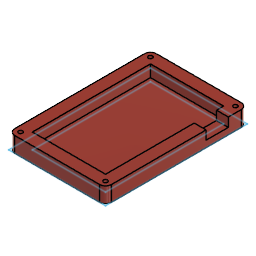
bottom_case (Autodesk Fusion 360 design; units mm, degrees)
part number: 2025-12-20-14-27-51-749
Autodesk Fusion 360 part; units mm, degrees
sketch "Schizzo1" plane through (0, 0, 0) normal (0, 0, 1) x (1, 0, 0)
  line L0 (11.1569, 43.4423) -> (72.6969, 43.4423)
  line L1 (72.6969, 43.4423) -> (72.6969, -55.9077)
  line L2 (72.6969, -55.9077) -> (11.1569, -55.9077)
  line L3 (11.1569, -55.9077) -> (11.1569, 43.4423)
  line L4 (1.157, 53.442) -> (82.697, 53.442)
  line L5 (82.697, 53.442) -> (82.697, -65.908)
  line L6 (82.697, -65.908) -> (1.157, -65.908)
  line L7 (1.157, -65.908) -> (1.157, 53.442)
  dimension "d1" = 99.35
  dimension "d2" = 61.54
  dimension "d3" = 81.54
  dimension "d4" = 119.35
  constraint horizontal L0
  constraint vertical L1
  constraint horizontal L2
  constraint vertical L3
  constraint horizontal L4
  constraint vertical L5
  constraint horizontal L6
  constraint vertical L7
  measures "d1" distance of L0.start L2.end
  measures "d2" distance of L1.end L2.end
  measures "d3" distance of L4.start L4.end
  measures "d4" distance of L4.start L6.end
sketch "Schizzo2" plane through (0, 0, 0) normal (0, 0, 1) x (1, 0, 0)
  circle A0 centre (6.1575, -60.9075) radius 1.7
  circle A1 centre (77.6967, -60.908) radius 1.7
  circle A2 centre (77.6975, 48.4425) radius 1.7
  circle A3 centre (6.1571, 48.442) radius 1.7
  circle A4 centre (6.1575, -60.9075) radius 3
  circle A5 centre (77.6967, -60.908) radius 3
  circle A6 centre (77.6975, 48.4425) radius 3
  circle A7 centre (6.1571, 48.442) radius 3
  dimension "d12" = 3.4
  dimension "d13" = 3.4
  dimension "d18" = 3.4
  dimension "d19" = 3.4
  dimension "d22" = 6
  dimension "d23" = 6
  dimension "d24" = 6
  dimension "d25" = 6
  constraint concentric A0 A4
  constraint concentric A1 A5
  constraint concentric A2 A6
  constraint concentric A3 A7
  measures "d12" diameter of A0
  measures "d13" diameter of A1
  measures "d18" diameter of A2
  measures "d19" diameter of A3
  measures "d22" diameter of A4
  measures "d23" diameter of A5
  measures "d24" diameter of A6
  measures "d25" diameter of A7
extrude "Estrusione1" add sketch "Schizzo2" along normal blind 9.9 from surface at 3.1 makes body 1 at (3.1608, 48.2924, 9.7) makes body 2 at (9.1538, -61.057, 9.7) makes body 3 at (76.3289, 45.7729, 6.4) makes body 4 at (76.3281, -63.5776, 6.4)
extrude "Estrusione2" add sketch "Schizzo1" along normal blind 13 bodies 1 2 3 4
extrude "Estrusione3" add sketch "Schizzo1" along normal blind 3 contours L0 L1 L2 L3 bodies 1
extrude "Estrusione4" cut sketch "Schizzo2" along normal blind 9.9 from surface at 3.1 contours A0 | A1 | A2 | A3 bodies 1
sketch "Schizzo3" plane through (0, 0, 13) normal (0, 0, 1) x (-1, 0, 0)
  circle A0 centre (-77.6975, -48.4425) radius 1.7
  circle A1 centre (-77.6967, 60.908) radius 1.7
  circle A2 centre (-6.1571, -48.442) radius 1.7
  circle A3 centre (-6.1575, 60.9075) radius 1.7
  line L0 (-72.6969, 55.9077) -> (-11.1569, 55.9077)
  line L1 (-11.1569, 55.9077) -> (-11.1569, -43.4423)
  line L2 (-11.1569, -43.4423) -> (-72.6969, -43.4423)
  line L3 (-72.6969, -43.4423) -> (-72.6969, 55.9077)
  line L4 (-1.157, 65.908) -> (-82.697, 65.908)
  line L5 (-82.697, 65.908) -> (-82.697, -53.442)
  line L6 (-82.697, -53.442) -> (-1.157, -53.442)
  line L7 (-1.157, -53.442) -> (-1.157, 65.908)
  line L8 (-82.697, -53.442) -> (-82.697, -37.492)
  line L9 (-82.697, -37.492) -> (-72.697, -37.492)
  line L10 (-72.697, -37.492) -> (-72.697, -18.742)
  line L11 (-72.697, -18.742) -> (-82.697, -18.742)
  line L12 (-82.697, -18.742) -> (-82.697, -37.492)
  dimension "d36" = 15.95
  dimension "d37" = 10
  dimension "d38" = 18.75
  constraint coincident L5.end L6.start
  constraint perpendicular L6 L8
  constraint horizontal L9
  constraint vertical L10
  constraint horizontal L11
  constraint vertical L12
  measures "d36" distance of L5.end L8.end
  measures "d37" distance of L8.end L9.end
  measures "d38" distance of L8.end L11.end
extrude "Estrusione5" cut sketch "Schizzo3" against normal blind 7.5 contours L3 L5 L9 L10 L11 L12 bodies 1
fillet "Raccordo1" radius 5 1 edges at (82.697, 53.442, 6.5) on bodies 1
fillet "Raccordo2" radius 5 1 edges at (82.697, -65.908, 6.5) on bodies 1
fillet "Raccordo3" radius 5 1 edges at (1.157, -65.908, 6.5) on bodies 1
fillet "Raccordo4" radius 5 1 edges at (1.157, 53.442, 6.5) on bodies 1
delete_face "EliminaFaccia1" 1 faces at (72.6972, 31.2422, 10.5001) on bodies 1
